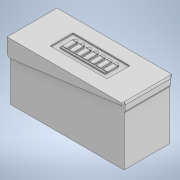
# Autodesk Inventor part: Ammo-Item-Medium
Saved by Autodesk Inventor 2020 (Build 240168000, 168)
## iProperties
Created: 2019-09-20
Part Number: Ammo-Item-Medium
Material: Generic
Document SubType Name: Modeling
Designer: vifly_01
Density: 1 g/cm^3
Appearance: Default
Author: vifly_01
Autodesk Inventor part; units mm, degrees
ref_plane "YZ Plane" through (0, 0, 0) normal (1, 0, 0) x (0, 1, 0)
ref_plane "XZ Plane" through (0, 0, 0) normal (0, 1, 0) x (-1, 0, 0)
ref_plane "XY Plane" through (0, 0, 0) normal (0, 0, 1) x (1, 0, 0)
sketch "Sketch1" plane through (0, 0, 0) normal (0, 0, 1) x (1, 0, 0)
  line L0 (-25, -10) -> (25, -10)
  line L1 (25, -10) -> (25, 10)
  line L2 (25, 10) -> (-25, 10)
  line L3 (-25, 10) -> (-25, -10)
  line L4 (-25, -10) -> (25, 10) construction
  line L5 (25, -10) -> (-25, 10) construction
  point P0 (0, 0)
  dimension "d0" = 50
  dimension "d1" = 20
  constraints: 12 end point, 2 midpoint, 2 parallel, 1 horizontal, 1 perpendicular
  measures "d0" distance of L2.end L1.end
  measures "d1" distance of L1.end L0.end
extrude "Extrusion1" add sketch "Sketch1" along normal blind 25
sketch "Sketch3" plane through (-25, -10, 0) normal (0, -1, 0) x (1, 0, 0)
  line L0 (0, 26) -> (50, 26)
  line L1 (50, 26) -> (50, 25)
  line L2 (50, 0) -> (50, 25) projected
  line L3 (50, 25) -> (1.2607, 18.4598)
  line L4 (0, 25) -> (50, 25) projected
  line L5 (0, 25) -> (50, 25)
  line L6 (0, 25) -> (-0.5, 25)
  line L7 (0, 26) -> (-0.5, 26)
  line L8 (-0.5, 26) -> (-0.5, 25)
  line L9 (-0.5, 25) -> (-0.5, 20)
  arc A0 (-0.5, 20) -> (1.2607, 18.4598) centre (1.054, 20) ccw
  point P0 (25, 0)
  dimension "d4" = 1
  dimension "d6" = 48.7393
  dimension "d12" = 0.5
  dimension "d13" = 5
  constraints: 16 end point, 2 horizontal, 2 perpendicular, 2 point on circle, 2 tangent, 1 centre point, 1 point on line, 1 vertical
  measures "d4" distance of L4.start L0.start
  measures "d6" horizontal distance of L1.end L3.end
  measures "d12" distance of L4.start L6.end
  measures "d13" distance of L6.end L9.end
extrude "Extrusion2" add sketch "Sketch3" along normal blind 1
extrude "Extrusion3" add sketch "Sketch3" against normal blind 21
sketch "Sketch4" plane through (-25.5, -11, 20) normal (-1, 0, 0) x (0, 0, 1)
  line L0 (-1.5402, 21) -> (5, 21) projected
  line L1 (5, 21) -> (-1.5402, 21)
  line L2 (-1.5402, 1) -> (-1.5402, 0) projected
  line L3 (-1.5402, 21) -> (-1.5402, 1)
  line L4 (-20, 1) -> (5, 1) projected
  line L5 (-1.5402, 1) -> (5, 1)
  line L6 (5, 1) -> (5, 21)
  point P0 (-20, 11)
  constraints: 8 end point, 2 collinear, 2 perpendicular
extrude "Extrusion4" cut sketch "Sketch4" against normal blind 0.5
sketch "Sketch5" plane through (25, -10, 0) normal (1, 0, 0) x (0, 0, -1)
  line L0 (-25, 0) -> (-18.4598, 0) projected
  line L1 (-18.4598, 20) -> (-25, 20) projected
  line L2 (-21.7299, 0) -> (-21.7299, 20)
  line L3 (-21.7299, 20) -> (-25, 20)
  line L4 (-25, 20) -> (-25, 0)
  line L5 (-25, 0) -> (-21.7299, 0)
  point P0 (0, 10)
  constraints: 8 end point, 2 midpoint, 2 parallel, 1 perpendicular
extrude "Extrusion5" add sketch "Sketch5" along normal blind 0.5
sketch "Sketch6" plane through (-25, -10, 0) normal (0, -1, 0) x (1, 0, 0)
  line L0 (50, 25) -> (50.5, 25) projected
  line L1 (50, 25) -> (50, 26) projected
  arc A0 (50.5, 25) -> (50, 26) centre (49.3829, 25.0664) ccw
  point P0 (25, 0)
  constraints: 2 point on circle, 1 centre point
extrude "Extrusion6" add sketch "Sketch6" against normal blind 20
sketch "Sketch7" plane through (-25, -10, 0) normal (0, -1, 0) x (1, 0, 0)
  line L0 (50, 21.7299) -> (50.5, 21.7299) projected
  line L1 (50, 21.7299) -> (50.5, 22.5959)
  line L2 (50.5, 21.7299) -> (50.5, 25) projected
  line L3 (50, 0) -> (50, 21.7299) projected
  line L4 (50, 21.7299) -> (50.5, 21.7299)
  line L5 (50.5, 21.7299) -> (50.5, 22.5959)
  point P0 (25, 0)
  dimension "d20" = 1
  constraints: 6 end point, 2 collinear, 1 point on line
  measures "d20" distance of L0.start L1.end
extrude "Extrusion7" cut sketch "Sketch7" against normal blind 20
sketch "Sketch11" plane through (-25.5, -11, 26) normal (0, 0, 1) x (1, 0, 0)
  line L0 (13, 6) -> (38, 6)
  line L1 (38, 6) -> (38, 16)
  line L2 (38, 16) -> (13, 16)
  line L3 (13, 16) -> (13, 6)
  line L4 (13, 6) -> (38, 16) construction
  line L5 (38, 6) -> (13, 16) construction
  line L6 (24.5, 8.75) -> (26.5, 8.75)
  line L7 (26.5, 8.75) -> (26.5, 13.25)
  line L8 (26.5, 13.25) -> (24.5, 13.25)
  line L9 (24.5, 13.25) -> (24.5, 8.75)
  line L10 (24.5, 8.75) -> (26.5, 13.25) construction
  line L11 (26.5, 8.75) -> (24.5, 13.25) construction
  line L12 (15.5, 8.5) -> (35.5, 8.5)
  line L13 (35.5, 8.5) -> (35.5, 7.75)
  line L14 (35.5, 7.75) -> (15.5, 7.75)
  line L15 (15.5, 7.75) -> (15.5, 8.5)
  line L16 (24.5, 13.35) -> (26.5, 13.35)
  arc A0 (26.5, 13.35) -> (24.5, 13.35) centre (25.5, 13.35) ccw
  line L17 (21.5, 13.25) -> (21.5, 8.75)
  line L18 (21.5, 8.75) -> (23.5, 8.75)
  line L19 (23.5, 13.25) -> (21.5, 13.25)
  line L20 (21.5, 8.75) -> (23.5, 13.25) construction
  line L21 (23.5, 8.75) -> (21.5, 13.25) construction
  line L22 (21.5, 13.35) -> (23.5, 13.35)
  arc A1 (23.5, 13.35) -> (21.5, 13.35) centre (22.5, 13.35) ccw
  line L23 (23.5, 8.75) -> (23.5, 13.25)
  line L24 (18.5, 13.25) -> (18.5, 8.75)
  line L25 (18.5, 8.75) -> (20.5, 8.75)
  line L26 (20.5, 13.25) -> (18.5, 13.25)
  line L27 (18.5, 8.75) -> (20.5, 13.25) construction
  line L28 (20.5, 8.75) -> (18.5, 13.25) construction
  line L29 (18.5, 13.35) -> (20.5, 13.35)
  arc A2 (20.5, 13.35) -> (18.5, 13.35) centre (19.5, 13.35) ccw
  line L30 (20.5, 8.75) -> (20.5, 13.25)
  line L31 (15.5, 13.25) -> (15.5, 8.75)
  line L32 (15.5, 8.75) -> (17.5, 8.75)
  line L33 (17.5, 13.25) -> (15.5, 13.25)
  line L34 (15.5, 8.75) -> (17.5, 13.25) construction
  line L35 (17.5, 8.75) -> (15.5, 13.25) construction
  line L36 (15.5, 13.35) -> (17.5, 13.35)
  arc A3 (17.5, 13.35) -> (15.5, 13.35) centre (16.5, 13.35) ccw
  line L37 (17.5, 8.75) -> (17.5, 13.25)
  line L38 (27.5, 13.25) -> (27.5, 8.75)
  line L39 (27.5, 8.75) -> (29.5, 8.75)
  line L40 (29.5, 13.25) -> (27.5, 13.25)
  line L41 (27.5, 8.75) -> (29.5, 13.25) construction
  line L42 (29.5, 8.75) -> (27.5, 13.25) construction
  line L43 (27.5, 13.35) -> (29.5, 13.35)
  arc A4 (29.5, 13.35) -> (27.5, 13.35) centre (28.5, 13.35) ccw
  line L44 (29.5, 8.75) -> (29.5, 13.25)
  line L45 (24.5, 13.25) -> (24.5, 8.75)
  line L46 (24.5, 8.75) -> (26.5, 8.75)
  line L47 (26.5, 13.25) -> (24.5, 13.25)
  line L48 (24.5, 8.75) -> (26.5, 13.25) construction
  line L49 (26.5, 8.75) -> (24.5, 13.25) construction
  line L50 (24.5, 13.35) -> (26.5, 13.35)
  arc A5 (26.5, 13.35) -> (24.5, 13.35) centre (25.5, 13.35) ccw
  line L51 (26.5, 8.75) -> (26.5, 13.25)
  line L52 (21.5, 13.25) -> (21.5, 8.75)
  line L53 (21.5, 8.75) -> (23.5, 8.75)
  line L54 (23.5, 13.25) -> (21.5, 13.25)
  line L55 (21.5, 8.75) -> (23.5, 13.25) construction
  line L56 (23.5, 8.75) -> (21.5, 13.25) construction
  line L57 (21.5, 13.35) -> (23.5, 13.35)
  arc A6 (23.5, 13.35) -> (21.5, 13.35) centre (22.5, 13.35) ccw
  line L58 (23.5, 8.75) -> (23.5, 13.25)
  line L59 (18.5, 13.25) -> (18.5, 8.75)
  line L60 (18.5, 8.75) -> (20.5, 8.75)
  line L61 (20.5, 13.25) -> (18.5, 13.25)
  line L62 (18.5, 8.75) -> (20.5, 13.25) construction
  line L63 (20.5, 8.75) -> (18.5, 13.25) construction
  line L64 (18.5, 13.35) -> (20.5, 13.35)
  arc A7 (20.5, 13.35) -> (18.5, 13.35) centre (19.5, 13.35) ccw
  line L65 (20.5, 8.75) -> (20.5, 13.25)
  line L66 (30.5, 13.25) -> (30.5, 8.75)
  line L67 (30.5, 8.75) -> (32.5, 8.75)
  line L68 (32.5, 13.25) -> (30.5, 13.25)
  line L69 (30.5, 8.75) -> (32.5, 13.25) construction
  line L70 (32.5, 8.75) -> (30.5, 13.25) construction
  line L71 (30.5, 13.35) -> (32.5, 13.35)
  arc A8 (32.5, 13.35) -> (30.5, 13.35) centre (31.5, 13.35) ccw
  line L72 (32.5, 8.75) -> (32.5, 13.25)
  line L73 (27.5, 13.25) -> (27.5, 8.75)
  line L74 (27.5, 8.75) -> (29.5, 8.75)
  line L75 (29.5, 13.25) -> (27.5, 13.25)
  line L76 (27.5, 8.75) -> (29.5, 13.25) construction
  line L77 (29.5, 8.75) -> (27.5, 13.25) construction
  line L78 (27.5, 13.35) -> (29.5, 13.35)
  arc A9 (29.5, 13.35) -> (27.5, 13.35) centre (28.5, 13.35) ccw
  line L79 (29.5, 8.75) -> (29.5, 13.25)
  line L80 (24.5, 13.25) -> (24.5, 8.75)
  line L81 (24.5, 8.75) -> (26.5, 8.75)
  line L82 (26.5, 13.25) -> (24.5, 13.25)
  line L83 (24.5, 8.75) -> (26.5, 13.25) construction
  line L84 (26.5, 8.75) -> (24.5, 13.25) construction
  line L85 (24.5, 13.35) -> (26.5, 13.35)
  arc A10 (26.5, 13.35) -> (24.5, 13.35) centre (25.5, 13.35) ccw
  line L86 (26.5, 8.75) -> (26.5, 13.25)
  line L87 (21.5, 13.25) -> (21.5, 8.75)
  line L88 (21.5, 8.75) -> (23.5, 8.75)
  line L89 (23.5, 13.25) -> (21.5, 13.25)
  line L90 (21.5, 8.75) -> (23.5, 13.25) construction
  line L91 (23.5, 8.75) -> (21.5, 13.25) construction
  line L92 (21.5, 13.35) -> (23.5, 13.35)
  arc A11 (23.5, 13.35) -> (21.5, 13.35) centre (22.5, 13.35) ccw
  line L93 (23.5, 8.75) -> (23.5, 13.25)
  line L94 (33.5, 13.25) -> (33.5, 8.75)
  line L95 (33.5, 8.75) -> (35.5, 8.75)
  line L96 (35.5, 13.25) -> (33.5, 13.25)
  line L97 (33.5, 8.75) -> (35.5, 13.25) construction
  line L98 (35.5, 8.75) -> (33.5, 13.25) construction
  line L99 (33.5, 13.35) -> (35.5, 13.35)
  arc A12 (35.5, 13.35) -> (33.5, 13.35) centre (34.5, 13.35) ccw
  line L100 (35.5, 8.75) -> (35.5, 13.25)
  line L101 (30.5, 13.25) -> (30.5, 8.75)
  line L102 (30.5, 8.75) -> (32.5, 8.75)
  line L103 (32.5, 13.25) -> (30.5, 13.25)
  line L104 (30.5, 8.75) -> (32.5, 13.25) construction
  line L105 (32.5, 8.75) -> (30.5, 13.25) construction
  line L106 (30.5, 13.35) -> (32.5, 13.35)
  arc A13 (32.5, 13.35) -> (30.5, 13.35) centre (31.5, 13.35) ccw
  line L107 (32.5, 8.75) -> (32.5, 13.25)
  line L108 (27.5, 13.25) -> (27.5, 8.75)
  line L109 (27.5, 8.75) -> (29.5, 8.75)
  line L110 (29.5, 13.25) -> (27.5, 13.25)
  line L111 (27.5, 8.75) -> (29.5, 13.25) construction
  line L112 (29.5, 8.75) -> (27.5, 13.25) construction
  line L113 (27.5, 13.35) -> (29.5, 13.35)
  arc A14 (29.5, 13.35) -> (27.5, 13.35) centre (28.5, 13.35) ccw
  line L114 (29.5, 8.75) -> (29.5, 13.25)
  line L115 (24.5, 13.25) -> (24.5, 8.75)
  line L116 (24.5, 8.75) -> (26.5, 8.75)
  line L117 (26.5, 13.25) -> (24.5, 13.25)
  line L118 (24.5, 8.75) -> (26.5, 13.25) construction
  line L119 (26.5, 8.75) -> (24.5, 13.25) construction
  line L120 (24.5, 13.35) -> (26.5, 13.35)
  arc A15 (26.5, 13.35) -> (24.5, 13.35) centre (25.5, 13.35) ccw
  line L121 (26.5, 8.75) -> (26.5, 13.25)
  point P0 (25.5, 11)
  point P1 (22.5, 11)
  point P2 (19.5, 11)
  point P3 (16.5, 11)
  point P4 (28.5, 11)
  point P5 (25.5, 11)
  point P6 (22.5, 11)
  point P7 (19.5, 11)
  point P8 (31.5, 11)
  point P9 (28.5, 11)
  point P10 (25.5, 11)
  point P11 (22.5, 11)
  point P12 (34.5, 11)
  point P13 (31.5, 11)
  point P14 (28.5, 11)
  point P15 (25.5, 11)
  dimension "d30" = 25
  dimension "d31" = 10
  dimension "d32" = 2
  dimension "d33" = 4.5
  dimension "d44" = 0.75
  dimension "d47" = 1
  dimension "d50" = 3
  dimension "d53" = 3
  constraints: 244 end point, 35 midpoint, 32 point on circle, 16 centre point, 16 point on line, 5 horizontal, 5 perpendicular, 4 parallel, 240 other
  measures "d30" distance of L2.end L1.end
  measures "d31" distance of L1.end L0.end
  measures "d32" distance of L8.end L7.end
  measures "d33" distance of L7.end L6.end
  measures "d44" distance of L12.end L13.end
  measures "d47" radius of A0
  measures "d50" distance of L6.start L17.end
  measures "d53" distance of L6.start L38.end
extrude "Extrusion10" cut sketch "Sketch11" against normal blind 0.5
body "Solid1"
